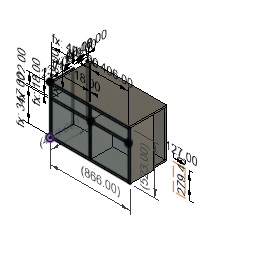
model (Autodesk Fusion 360 design; units mm, degrees)
Autodesk Fusion 360 part; units mm, degrees
sketch "Sketch1" plane through (0, 0, 0) normal (0, 1, 0) x (1, 0, 0)
  line L0 (0, 0) -> (866, 0)
  line L1 (866, 0) -> (866, -523)
  line L2 (866, -523) -> (0, -523)
  line L3 (0, -523) -> (0, 0)
  line L4 (848, -505) -> (18, -505)
  line L5 (18, -505) -> (18, -18)
  line L6 (18, -18) -> (848, -18)
  line L7 (848, -18) -> (848, -505)
  line L8 (433, -18) -> (433, -505) construction
  line L9 (424, -505) -> (424, -18)
  line L10 (442, -18) -> (442, -505)
  line L11 (424, -505) -> (442, -18) construction
  line L12 (18, -383) -> (424, -383)
  line L13 (18, -365) -> (424, -365)
  line L14 (848, -365) -> (442, -365)
  line L15 (848, -383) -> (442, -383)
  line L16 (18, -505) -> (18, -523)
  line L17 (848, -505) -> (848, -523)
  line L18 (848, -18) -> (848, 0)
  line L19 (18, -18) -> (18, 0)
  line L20 (1333.7188, -442.8997) -> (1460.7188, -442.8997) construction
  line L21 (1460.7188, -442.8997) -> (1460.7188, -163.4997) construction
  line L22 (1460.7188, -163.4997) -> (1333.7188, -163.4997) construction
  line L23 (1333.7188, -163.4997) -> (1333.7188, -442.8997) construction
  dimension "d2" = 18
  dimension "d3" = 18
  dimension "d4" = 406
  dimension "d5" = 406
  dimension "d7" = 18
  dimension "d8" = 347
  dimension "d9" = 122
  dimension "d10" = 523
  dimension "d12" = 127
  dimension "d13" = 279.4
  dimension "d14" = 866
  constraint horizontal L0
  constraint vertical L1
  constraint horizontal L2
  constraint vertical L3
  constraint coincident L0.start L3.end
  constraint midpoint L6 L8.start
  constraint midpoint L4 L8.end
  constraint perpendicular L4 L8
  constraint coincident L4 L9.start
  constraint coincident L6 L9.end
  constraint coincident L6 L10.start
  constraint coincident L4 L10.end
  constraint vertical L9
  constraint vertical L10
  constraint midpoint L8 L11
  constraint coincident L5 L12.start
  constraint coincident L9 L12.end
  constraint coincident L5 L13.start
  constraint coincident L9 L13.end
  constraint horizontal L13
  constraint horizontal L12
  constraint symmetric L8 L12.start L15.start
  constraint symmetric L8 L12.end L15.end
  constraint symmetric L8 L13.start L14.start
  constraint symmetric L8 L13.end L14.end
  constraint coincident L2 L16.end
  constraint coincident L2 L17.end
  constraint coincident L0 L18.end
  constraint coincident L0 L19.end
  constraint vertical L19
  constraint vertical L16
  constraint vertical L17
  constraint vertical L18
  constraint horizontal L20
  constraint vertical L21
  constraint horizontal L22
  constraint vertical L23
  measures "d3" distance of L9.start L10.end
  measures "d4" distance of L4.end L9.start
  measures "d5" distance of L4.start L10.end
  measures "d7" distance of L12.start L13.start
  measures "d8" distance of L5.end L13.start
  measures "d9" distance of L4.end L12.start
  measures "d10" distance of L0.end L1.end
  measures "d12" distance of L20.start L20.end
  measures "d13" distance of L20.end L21.end
  measures "d14" distance of L0.start L0.end
sketch "Sketch2" plane through (0, 0, 0) normal (1, 0, 0) x (0, 1, 0)
  line L0 (0, 523) -> (255, 523)
  line L1 (255, 523) -> (255, 0)
  line L2 (255, 0) -> (0, 0)
  line L3 (0, 0) -> (0, 523)
  line L4 (237, 523) -> (237, 0)
  line L5 (413, 0) -> (395, 0)
  line L6 (395, 0) -> (395, 523)
  line L7 (395, 523) -> (413, 523)
  line L8 (413, 523) -> (413, 0)
  point P0 (0, 523)
  dimension "d15" = 18
  dimension "d16" = 237
  dimension "d17" = 18
  dimension "d18" = 140
  dimension "d19" = 413
  constraint horizontal L0
  constraint vertical L1
  constraint horizontal L2
  constraint vertical L3
  constraint coincident P0 L0.start
  constraint coincident L2.end L3.start
  constraint coincident L0 L4.start
  constraint coincident L2 L4.end
  constraint vertical L4
  constraint horizontal L5
  constraint vertical L6
  constraint horizontal L7
  constraint vertical L8
  constraint equal L1 L6
  constraint collinear L2 L5
  measures "d15" distance of L0.end L4.start
  measures "d16" distance of P0 L4.start
  measures "d17" distance of L6.end L7.end
  measures "d18" distance of L0.end L6.end
  measures "d19" distance of L5.start L2.end
extrude "Extrude1" add sketch "Sketch1" along normal up to surface (413 mm away) contours L0 L6 L18 L19 | L2 L4 L16 L17 makes body 1 at (294.6667, 137.6667, 0) makes body 2 at (294.6667, 275.3333, 523)
extrude "Extrude5" add sketch "Sketch1" along normal up to surface (237 mm away) separate body contours L5 L9 L12 L13 | L7 L10 L14 L15 makes body 3 at (712.6667, 79, 383) makes body 4 at (153.3333, 79, 365)
extrude "Extrude2" add sketch "Sketch1" along normal up to surface (255 mm away) separate body contours L0 L2 L3 L5 L16 L19 | L0 L1 L2 L7 L17 L18 | L4 L6 L9 L10 makes body 5 at (866, 170, 174.3333) makes body 6 at (442, 85, 180.3333) makes body 7 at (18, 85, 348.6667)
extrude "Extrude3" add sketch "Sketch2" along normal up to surface (830 mm away) from surface at 18 separate body contours L5 L6 L7 L8 makes body 8
extrude "Extrude4" add sketch "Sketch2" along normal up to surface (830 mm away) from surface at 18 separate body contours L0 L1 L2 L4 makes body 9
combine "Combine1" operation cut target body 6 tool bodies 9 keep tools
combine "Combine2" operation cut target body 9 tool bodies 2 1 keep tools
combine "Combine3" operation cut target body 8 tool bodies 2 1 keep tools
equation "th = 18 mm"
equation "d2 = th"
equation "d3 = th"
equation "d4 = 396 mm + margin"
equation "d5 = d4"
equation "d7 = th"
equation "d8 = 337 mm + margin"
equation "d9 = 112 mm + margin"
equation "margin = 10 mm"
equation "d12 = 5\""
equation "d13 = 11\""
equation "d15 = th"
equation "d17 = th"
